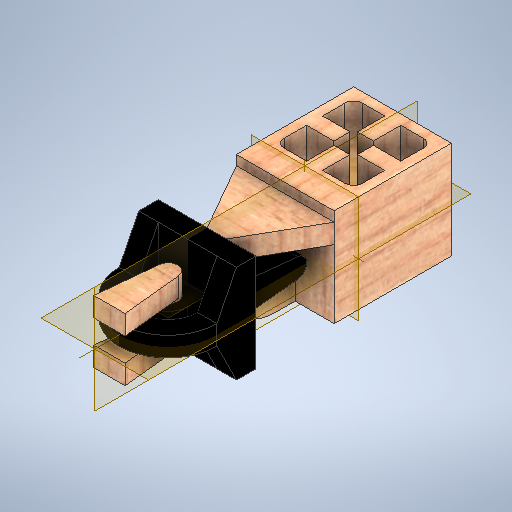
# Autodesk Inventor part: SoporteCamara
Saved by Autodesk Inventor 2025.2 (Build 292293000, 293)
## iProperties
Created: 2025-03-24
Part Number: SoporteCamara
Material: Genérico
Document SubType Name: Modeling
Designer: braug
Density: 1 g/cm^3
Appearance: Abedul - Natural pulido
Author: braug
## iProperties of the stored document SoporteCamara_3DPrint.ipt
Created: 2025-03-25
Part Number: SoporteCamara_3DPrint
Material: Genérico
Document SubType Name: Modeling
Designer: braug
Density: 1 g/cm^3
Appearance: Valor por defecto
Author: braug
Autodesk Inventor part; units mm, degrees
sketch "Boceto1" plane through (0, 0, 0) normal (0, 0, 1) x (1, 0, 0)
  line L0 (-25, -25) -> (25, -25)
  line L1 (25, -25) -> (25, 25)
  line L2 (25, 25) -> (-25, 25)
  line L3 (-25, 25) -> (-25, -25)
  line L4 (-25, -25) -> (25, 25) construction
  line L5 (25, -25) -> (-25, 25) construction
  point P0 (0, 0)
  dimension "d0" = 50
  dimension "d1" = 50
  constraints: 12 end point, 2 midpoint, 2 parallel, 1 horizontal, 1 perpendicular
  measures "d0" distance of L2.end L1.end
  measures "d1" distance of L1.end L0.end
extrude "Extrusión1" add sketch "Boceto1" along normal blind 10
sketch "Boceto2" plane through (0, 0, 0) normal (1, 0, 0) x (0, 1, 0)
  line L0 (-25, 10) -> (25, 10) projected
  line L1 (-10, 20) -> (-10, 10)
  arc A0 (0, 30) -> (-10, 20) centre (0, 20) ccw
  arc A1 (0, 35) -> (-15, 20) centre (0, 20) ccw
  line L2 (-15, 20) -> (-15, 10)
  arc A2 (0, 45) -> (-25, 20) centre (0, 20) ccw
  line L3 (-25, 20) -> (-25, 10)
  line L4 (-25, 10) -> (0, 10)
  circle A3 centre (0, 20) radius 5.2
  line L5 (0, 30) -> (10, 30)
  line L6 (10, 30) -> (10, 31.1803)
  line L7 (10, 35) -> (0, 35)
  line L8 (0, 45) -> (10, 45)
  line L9 (10, 45) -> (10, 35)
  line L10 (10, 30) -> (10, 10)
  line L11 (10, 10) -> (0, 10)
  point P0 (0, 0)
  dimension "d17" = 20
  dimension "d18" = 25
  dimension "d20" = 10
  dimension "d21" = 10
  dimension "d26" = 10.4
  dimension "d27" = 10
  dimension "d28" = 35
  constraints: 22 end point, 7 point on circle, 5 point on line, 4 centre point, 3 coincident, 3 perpendicular, 3 tangent, 2 collinear, 1 horizontal, 1 midpoint, 1 parallel
  measures "d17" distance of L5.start L4.end
  measures "d18" distance of L7.end L4.end
  measures "d20" distance of L3.start L0.start
  measures "d21" distance of L4.end A2.centre
  measures "d26" diameter of A3
  measures "d27" distance of L5.start L5.end
  measures "d28" distance of L10.end L8.end
extrude "Extrusión2" add sketch "Boceto2" along normal mid plane 10
sketch "Boceto5" plane through (-5, 10, 30) normal (0, 1, 0) x (1, 0, 0)
  line L0 (30, 20) -> (-20, 20) projected
  line L1 (0, 10) -> (0, -15) projected
  line L2 (-20, 20) -> (0, -15)
  line L3 (0, -15) -> (9.9814, -15)
  line L4 (9.9814, -15) -> (30, 20)
  line L5 (30, 20) -> (-20, 20)
  point P0 (5, 30)
  constraints: 8 end point, 1 parallel, 1 perpendicular
extrude "Extrusión4" add sketch "Boceto5" along normal blind 10
ref_plane "Plano de trabajo2" through (6, 0, 0) normal (1, 0, 0) x (0, 0, -1)
sketch "Boceto6" plane through (6, 0, 0) normal (1, 0, 0) x (0, 0, -1)
  circle A0 centre (-20, 0) radius 5.2 projected
  circle A1 centre (-20, 0) radius 5
  arc A2 (-35, 0) -> (-20, -15) centre (-20, 0) ccw projected
  arc A3 (-30, 0) -> (-20, -10) centre (-20, 0) ccw projected
  line L0 (-35, 0) -> (-30, 0) construction
  circle A4 centre (-32.5, 0) radius 2.3
  point P0 (0, 0)
  dimension "d32" = 10
  dimension "d33" = 4.6
  constraints: 2 centre point, 2 end point, 1 coincident, 1 horizontal, 1 midpoint
  measures "d32" diameter of A1
  measures "d33" diameter of A4
extrude "Extrusión5" add sketch "Boceto6" against normal blind 12 contours A1 | A4
sketch "Boceto7" plane through (6, 0, 0) normal (1, 0, 0) x (0, 0, -1)
  line L0 (0, 0) -> (-64.0101, 0) construction
  circle A0 centre (-20, 0) radius 5 projected
  arc A1 (-15, 0) -> (-19.5073, 4.9757) centre (-20, 0) ccw
  line L1 (-45, 10) -> (-45, 0) projected
  line L2 (-45, 10) -> (-45, 7.5)
  line L3 (-45, 7.5) -> (-19.5073, 4.9757)
  arc A2 (-45, 0) -> (-20, -25) centre (-20, 0) ccw projected
  line L4 (-45, 0) -> (-45, 7.5)
  line L5 (-45, 0) -> (-50, 0)
  line L6 (-50, 0) -> (-50, 10)
  line L7 (-19.5073, 4.9757) -> (-50, 7.9951)
  arc A3 (-19.5073, -4.9757) -> (-15, 0) centre (-20, 0) ccw
  line L8 (-50, 0) -> (-50, -10)
  line L9 (-19.5073, -4.9757) -> (-50, -7.9951)
  dimension "d36" = 10
  dimension "d37" = 2.5
  dimension "d38" = 5
  constraints: 18 end point, 6 point on line, 4 point on circle, 3 symmetric about line, 2 centre point, 1 coincident, 1 collinear, 1 horizontal, 1 perpendicular, 1 tangent, 1 other
  measures "d36" diameter of A1
  measures "d37" distance of L1.start L2.end
  measures "d38" distance of L1.end L5.end
extrude "Extrusión6" add sketch "Boceto7" along normal blind 10
sketch "Boceto8" plane through (-6, 0, 20) normal (-1, 0, 0) x (0, 0, 1)
  circle A0 centre (12.5, 0) radius 2.3 projected
  arc A1 (-0.4927, -4.9757) -> (-0.4927, 4.9757) centre (0, 0) ccw projected
  line L0 (30, -7.9951) -> (-0.4927, -4.9757) projected
  line L1 (30, 7.9951) -> (30, -7.9951) projected
  line L2 (-0.4927, 4.9757) -> (30, 7.9951) projected
  circle A2 centre (0, 0) radius 5 projected
  point P0 (-20, 0)
extrude "Extrusión7" add sketch "Boceto8" along normal blind 10 contours A0 | A2 A1 | A1 L2 L1 L0
sketch "Boceto9" plane through (6, -7.9951, 50) normal (0, 0, 1) x (1, 0, 0)
  line L0 (19, -17.0049) -> (19, 17.9951) projected
  line L1 (-31, -17.0049) -> (-11, -17.0049) projected
  line L2 (-31, 17.9951) -> (-31, -17.0049) projected
  line L3 (-11, -17.0049) -> (-1, -17.0049) projected
  line L4 (-1, -17.0049) -> (19, -17.0049) projected
  line L5 (-31, 27.9951) -> (-31, 17.9951) projected
  line L6 (19, 32.9951) -> (-31, 32.9951) projected
  line L7 (-31, 32.9951) -> (-31, 27.9951) projected
  line L8 (19, 27.9951) -> (19, 32.9951) projected
  line L9 (19, 17.9951) -> (19, 27.9951) projected
  point P0 (-6, 7.9951)
extrude "Extrusión8" add sketch "Boceto9" along normal blind 10
sketch "Boceto10" plane through (0, 0, 0) normal (0, 1, 0) x (-1, 0, 0)
  arc A0 (10, 70) -> (0, 80) centre (0, 70) ccw
  arc A1 (15, 70) -> (0, 85) centre (0, 70) ccw
  arc A2 (25, 70) -> (0, 95) centre (0, 70) ccw
  line L0 (10, 70) -> (10, 60)
  line L1 (15, 60) -> (15, 70)
  line L2 (25, 70) -> (25, 60)
  line L3 (25, 60) -> (15, 60)
  line L4 (10, 60) -> (0, 60)
  line L5 (0, 70) -> (0, 50)
  line L6 (0, 50) -> (0, 99.3046) construction
  line L7 (-10, 70) -> (-10, 60)
  line L8 (-10, 60) -> (0, 60)
  line L9 (-15, 60) -> (-15, 70)
  arc A3 (0, 80) -> (-10, 70) centre (0, 70) ccw
  line L10 (-25, 70) -> (-25, 60)
  line L11 (-25, 60) -> (-15, 60)
  arc A4 (0, 85) -> (-15, 70) centre (0, 70) ccw
  arc A5 (0, 95) -> (-25, 70) centre (0, 70) ccw
  line L12 (25, 60) -> (-25, 60) projected
  circle A6 centre (0, 70) radius 5.2
  point P0 (0, 0)
  point P1 (0, 72.5)
  point P2 (0, 67.5)
  point P3 (0, 60)
  dimension "d144" = 10
  dimension "d145" = 25
  dimension "d146" = 15
  dimension "d147" = 10
  dimension "d148" = 10.4
  constraints: 24 end point, 12 point on circle, 7 centre point, 7 coincident, 6 symmetric about line, 4 point on line, 1 midpoint, 1 parallel, 1 perpendicular, 1 vertical, 3 other
  measures "d144" distance of L10.start L10.end
  measures "d145" radius of A5
  measures "d146" radius of A1
  measures "d147" radius of A0
  measures "d148" diameter of A6
extrude "Extrusión9" add sketch "Boceto10" along normal mid plane 10 contours L0 L4 L8 L7 A3 A0 | L1 A1 A4 L9 L11 L10 A5 A2 L2 L3
ref_plane "Plano de trabajo3" through (0, 6, 0) normal (0, 1, 0) x (1, 0, 0)
sketch "Boceto11" plane through (0, 6, 0) normal (0, 1, 0) x (1, 0, 0)
  circle A0 centre (0, -70) radius 5
  arc A1 (-10, -70) -> (10, -70) centre (0, -70) ccw projected
  line L0 (0, -80) -> (0, -85)
  arc A2 (-15, -70) -> (15, -70) centre (0, -70) ccw projected
  circle A3 centre (0, -82.5) radius 2.3
  point P0 (0, 0)
  dimension "d57" = 10
  dimension "d58" = 4.6
  constraints: 2 centre point, 2 end point, 2 point on circle, 1 coincident, 1 midpoint, 1 vertical
  measures "d57" diameter of A0
  measures "d58" diameter of A3
extrude "Extrusión10" add sketch "Boceto11" against normal blind 12
sketch "Boceto13" plane through (-25, -25, 50) normal (-1, 0, 0) x (0, 0, 1)
  line L0 (0, 50) -> (0, 0) projected
  line L1 (0, 0) -> (10, 0) projected
  line L2 (10, 20) -> (10, 0) projected
  line L3 (20, 20) -> (10, 20) projected
  line L4 (20, 20) -> (20, 30) projected
  line L5 (10, 30) -> (20, 30) projected
  line L6 (10, 50) -> (10, 30) projected
  line L7 (0, 50) -> (10, 50) projected
  line L8 (20, 20) -> (10, 0)
  line L9 (10, 50) -> (20, 30)
  point P0 (-50, 25)
  point P1 (20, 20)
  point P2 (10, 20)
  constraints: 4 end point
extrude "Extrusión11" add sketch "Boceto13" against normal blind 10 contours L9 L5 L6 | L2 L3 L8
sketch "Boceto14" plane through (25, -25, 50) normal (1, 0, 0) x (0, 0, -1)
  line L0 (0, 0) -> (0, 50) projected
  line L1 (0, 50) -> (-10, 50) projected
  line L2 (-10, 30) -> (-10, 50) projected
  line L3 (-20, 30) -> (-10, 30) projected
  line L4 (-20, 20) -> (-20, 30) projected
  line L5 (-10, 20) -> (-20, 20) projected
  line L6 (-10, 0) -> (-10, 20) projected
  line L7 (0, 0) -> (-10, 0) projected
  line L8 (-10, 50) -> (-20, 30) projected
  line L9 (-20, 20) -> (-10, 0) projected
  point P0 (50, 25)
extrude "Extrusión12" add sketch "Boceto14" against normal blind 10 contours L9 L5 L6 | L2 L3 L8
sketch "Boceto15" plane through (-25, 25, 0) normal (0, 1, 0) x (1, 0, 0)
  line L0 (50, 0) -> (0, 0) projected
  line L1 (0, 0) -> (50, 0)
  line L2 (50, 0) -> (50, 50)
  line L3 (50, 50) -> (0, 50)
  line L4 (0, 50) -> (0, 0)
  line L5 (50, 0) -> (0, 50) construction
  line L6 (9.5, 5) -> (40.5, 5)
  line L7 (45, 9.5) -> (45, 40.5)
  line L8 (40.5, 45) -> (9.5, 45)
  line L9 (5, 40.5) -> (5, 9.5)
  line L10 (5, 5) -> (45, 45) construction
  line L11 (45, 5) -> (5, 45) construction
  arc A0 (5, 9.5) -> (9.5, 5) centre (9.2985, 9.2985) ccw
  line L12 (50, 50) -> (12.682, 12.682) construction
  line L13 (9.2985, 9.2985) -> (0, 0) construction
  line L14 (-9.6582, 130.7458) -> (57.4478, 130.7458) construction
  line L15 (57.4478, 130.7458) -> (57.4478, 74.9632) construction
  line L16 (57.4478, 74.9632) -> (-9.6582, 74.9632) construction
  line L17 (-9.6582, 74.9632) -> (-9.6582, 130.7458) construction
  circle A1 centre (25, 25) radius 3.4
  line L18 (20.4142, 19) -> (29.5858, 19)
  line L19 (31, 20.4142) -> (31, 29.5858)
  line L20 (29.5858, 31) -> (20.4142, 31)
  line L21 (19, 29.5858) -> (19, 20.4142)
  line L22 (19.6, 19.6) -> (30.4, 30.4) construction
  line L23 (30.4, 19.6) -> (19.6, 30.4) construction
  line L24 (20.4142, 31) -> (15.0142, 36.4)
  line L25 (35.25, 48.8) -> (14.75, 41.2) construction
  line L26 (14.75, 48.8) -> (35.25, 41.2) construction
  line L27 (15.0142, 45) -> (15.0142, 36.4)
  line L28 (13.7142, 37.7) -> (13.7142, 45)
  line L29 (5, 34.9858) -> (13.6, 34.9858)
  line L30 (12.3, 36.2858) -> (5, 36.2858)
  line L31 (19, 29.5858) -> (13.6, 34.9858)
  arc A2 (12.3, 36.2858) -> (13.7142, 37.7) centre (12.3, 37.7) ccw
  arc A3 (45, 40.5) -> (40.5, 45) centre (40.7015, 40.7015) ccw
  line L32 (25, 75.7962) -> (25, -2.7787) construction
  arc A4 (40.5, 5) -> (45, 9.5) centre (40.7015, 9.2985) ccw
  arc A5 (9.5, 45) -> (5, 40.5) centre (9.2985, 40.7015) ccw
  line L33 (31, 20.4142) -> (36.4, 15.0142)
  line L34 (45, 15.0142) -> (36.4, 15.0142)
  line L35 (37.7, 13.7142) -> (45, 13.7142)
  line L36 (34.9858, 5) -> (34.9858, 13.6)
  line L37 (36.2858, 12.3) -> (36.2858, 5)
  line L38 (29.5858, 19) -> (34.9858, 13.6)
  arc A6 (37.7, 13.7142) -> (36.2858, 12.3) centre (37.7, 12.3) ccw
  line L39 (29.5858, 31) -> (34.9858, 36.4)
  line L40 (34.9858, 45) -> (34.9858, 36.4)
  line L41 (36.2858, 37.7) -> (36.2858, 45)
  line L42 (45, 34.9858) -> (36.4, 34.9858)
  line L43 (37.7, 36.2858) -> (45, 36.2858)
  line L44 (31, 29.5858) -> (36.4, 34.9858)
  arc A7 (36.2858, 37.7) -> (37.7, 36.2858) centre (37.7, 37.7) ccw
  line L45 (13.7142, 12.3) -> (13.7142, 5)
  line L46 (15.0142, 5) -> (15.0142, 13.6)
  line L47 (20.4142, 19) -> (15.0142, 13.6)
  line L48 (19, 20.4142) -> (13.6, 15.0142)
  line L49 (5, 15.0142) -> (13.6, 15.0142)
  arc A8 (13.7142, 12.3) -> (12.3, 13.7142) centre (12.3, 12.3) ccw
  line L50 (12.3, 13.7142) -> (5, 13.7142)
  line L51 (36.2858, 37.7) -> (36.2858, 43.2358)
  line L52 (36.2858, 43.2358) -> (40.7015, 43.2358)
  line L53 (43.2358, 40.7015) -> (43.2358, 36.2858)
  line L54 (43.2358, 36.2858) -> (37.7, 36.2858)
  line L55 (6.7642, 13.7142) -> (6.7642, 6.7642)
  line L56 (6.7642, 6.7642) -> (13.7142, 6.7642)
  line L57 (13.7142, 43.2358) -> (6.7642, 43.2358)
  line L58 (6.7642, 43.2358) -> (6.7642, 36.2858)
  line L59 (43.2358, 13.7142) -> (43.2358, 6.7642)
  line L60 (43.2358, 6.7642) -> (36.2858, 6.7642)
  arc A9 (43.2358, 40.7015) -> (40.7015, 43.2358) centre (40.7015, 40.7015) ccw
  line L61 (29.1, 31.9873) -> (29.1, 45)
  line L62 (29.1, 45) -> (20.9, 45)
  line L63 (20.9, 45) -> (20.9, 31.9873)
  line L64 (20.9, 45) -> (20.9, 31)
  line L65 (29.1, 45) -> (29.1, 31)
  line L66 (5, 29.1) -> (19, 29.1)
  line L67 (5, 20.9) -> (19, 20.9)
  line L68 (45, 20.9) -> (31, 20.9)
  line L69 (45, 29.1) -> (31, 29.1)
  line L70 (29.1, 5) -> (29.1, 19)
  line L71 (20.9, 5) -> (20.9, 19)
  point P0 (25, 0)
  point P1 (25, 45)
  point P2 (43.2358, 43.2358)
  point P3 (25, 38.4937)
  point P4 (31.9873, 20.9)
  point P5 (20.9, 19)
  point P6 (20.9, 5)
  point P7 (19, 20.9)
  point P8 (19, 29.1)
  point P9 (31, 29.1)
  point P10 (45, 20.9)
  point P11 (29.1, 19)
  dimension "d66" = 50
  dimension "d67" = 50
  dimension "d68" = 40
  dimension "d69" = 40
  dimension "d89" = 6.8
  dimension "d93" = 1
  dimension "d94" = 20.5
  dimension "d96" = 1.3
  dimension "d106" = 6.95
  dimension "d107" = 6.95
  dimension "d108" = 14
  dimension "d109" = 14
  dimension "d110" = 40
  dimension "d115" = 8.2
  constraints: 134 end point, 67 symmetric about line, 18 point on circle, 12 parallel, 12 point on line, 10 centre point, 7 midpoint, 6 perpendicular, 3 coincident, 3 horizontal, 3 vertical, 1 tangent, 8 other
  measures "d66" distance of L3.end L2.end
  measures "d67" distance of L2.end L1.end
  measures "d68" distance of L11.end L10.end
  measures "d69" distance of L10.end L11.start
  measures "d89" diameter of A1
  measures "d93" distance between parallel lines of L11 L24
  measures "d94" distance of L26.end L25.end
  measures "d96" distance between parallel lines of L28 L27
  measures "d106" distance of L51.end point (43.236, 43.236)
  measures "d107" distance between parallel lines of L54 L52
  measures "d108" distance between parallel lines of L8 L20
  measures "d109" distance between parallel lines of L6 L18
  measures "d110" distance between parallel lines of L6 L8
  measures "d115" distance of L62.end L61.end
extrude "Extrusión15" add sketch "Boceto15" against normal up to surface (50 mm away) contours L0 L4 L3 L2 | L71 L18 L70 L6 | L9 L66 L21 L67 | L68 L19 L69 L7 | L8 L61 L65 L20 L64 L63
sketch "Boceto16" plane through (0, -6, 82.5) normal (0, -1, 0) x (1, 0, 0)
  arc A0 (0, -17.5) -> (4.9757, -12.9927) centre (0, -12.5) ccw
  line L0 (7.5, 12.5) -> (4.9757, -12.9927)
  line L1 (0, 17.5) -> (7.9951, 17.5)
  line L2 (4.9757, -12.9927) -> (7.9951, 17.5)
  line L3 (0, 17.5) -> (-7.9951, 17.5)
  line L4 (-4.9757, -12.9927) -> (-7.9951, 17.5)
  arc A1 (-4.9757, -12.9927) -> (0, -17.5) centre (0, -12.5) ccw
  circle A2 centre (0, 0) radius 2.3 projected
  line L5 (27.3818, -12.5) -> (-15.7186, -12.5) construction
  line L6 (0, -25.6017) -> (0, 0) construction
  point P0 (0, -82.5)
  point P1 (0, -12.5)
  point P2 (0, -12.5)
  dimension "d70" = 10
  constraints: 14 end point, 4 point on circle, 2 centre point, 1 coincident, 1 point on line, 1 tangent, 2 other
  measures "d70" diameter of A0
extrude "Extrusión13" add sketch "Boceto16" along normal blind 10 contours A1 L4 L3 L1 L2 L0 A0 | A2
sketch "Boceto17" plane through (0, 6, 70) normal (0, 1, 0) x (1, 0, 0)
  line L0 (7.9951, -30) -> (-7.9951, -30) projected
  line L1 (4.9757, 0.4927) -> (7.9951, -30) projected
  line L2 (-7.9951, -30) -> (-4.9757, 0.4927) projected
  arc A0 (-4.9757, 0.4927) -> (4.9757, 0.4927) centre (0, 0) ccw projected
  circle A1 centre (0, 0) radius 5 projected
  point P0 (0, 70)
extrude "Extrusión14" add sketch "Boceto17" along normal blind 10
fillet "Empalme15" [suppressed]
fillet "Empalme16" [suppressed]
fillet "Empalme17" [suppressed]
fillet "Empalme18" [suppressed]
fillet "Empalme19" [suppressed]
fillet "Empalme21" [suppressed]
fillet "Empalme22" [suppressed]
fillet "Empalme23" [suppressed]
